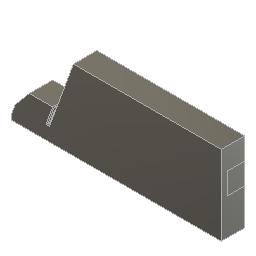
yomamamapHolder v6 (Autodesk Fusion 360 design; units mm, degrees)
Autodesk Fusion 360 part; units mm, degrees
sketch "Sketch1" plane through (0, 0, 0) normal (0, 0, 1) x (1, 0, 0)
  line L0 (0, 0) -> (12.2417, 33.6337)
  line L1 (0, 0) -> (48.7528, 0) construction
  line L2 (0, 0) -> (79.9419, 0)
  line L3 (0, 0) -> (-15, 0)
  line L4 (-1.62, 0) -> (2.6109, 11.6242)
  line L5 (-15, 0) -> (-15, -1)
  line L6 (-15, -1) -> (79.9419, -1)
  line L7 (79.9419, -1) -> (79.9419, 0)
  line L8 (2.059, 5.657) -> (2.9619, 8.1378)
  line L9 (2.9619, 8.1378) -> (18.5044, 2.4808)
  line L10 (18.5044, 2.4808) -> (17.6015, 0)
  line L11 (17.6015, 0) -> (2.059, 5.657)
  line L12 (2.9619, 8.1378) -> (3.3039, 9.0775)
  line L13 (3.3039, 9.0775) -> (17.9068, 3.7625)
  line L14 (17.9068, 3.7625) -> (17.5647, 2.8228)
  line L15 (17.5647, 2.8228) -> (2.9619, 8.1378)
  line L16 (1.717, 4.7173) -> (14.6777, 0)
  line L17 (1.546, 4.2475) -> (-13.454, 4.2475)
  line L18 (-15, 0) -> (-13.454, 4.2475)
  line L19 (12.9419, 32.6337) -> (78.9419, 32.6337)
  line L20 (78.9419, 32.6337) -> (78.9419, 6.6337)
  line L21 (78.9419, 6.6337) -> (12.9419, 6.6337)
  line L22 (12.9419, 6.6337) -> (12.9419, 32.6337)
  line L23 (12.2417, 33.6337) -> (79.9419, 33.6337)
  line L24 (79.9419, 33.6337) -> (79.9419, 0)
  line L25 (2.6109, 11.6242) -> (-7.2642, 11.6242)
  line L26 (-7.2642, 11.6242) -> (-13.454, 4.2475)
  line L27 (-8.6415, 4.2475) -> (-3.2666, 4.2475)
  line L28 (-3.2666, 4.2475) -> (-3.2666, 0)
  line L29 (-3.2666, 0) -> (-8.6415, 0)
  line L30 (-8.6415, 0) -> (-8.6415, 4.2475)
  line L31 (-3.2666, 4.2475) -> (-0.9456, 10.6242)
  line L32 (-0.9456, 10.6242) -> (1.8734, 9.5982)
  line L33 (-12.3719, 1) -> (-13.2911, 1.7713)
  line L34 (-13.2911, 1.7713) -> (-10.5662, 5.0188)
  line L35 (-10.5662, 5.0188) -> (-9.6469, 4.2475)
  line L36 (-9.6469, 4.2475) -> (-12.3719, 1)
  line L37 (12.7419, 15.4337) -> (11.7419, 15.4337)
  line L38 (11.7419, 15.4337) -> (11.7419, 5.4337)
  line L39 (11.7419, 5.4337) -> (21.7419, 5.4337)
  line L40 (21.7419, 5.4337) -> (21.7419, 6.4337)
  line L41 (12.7419, 15.4337) -> (12.7419, 6.4337)
  line L42 (12.7419, 6.4337) -> (21.7419, 6.4337)
  line L43 (59.9419, 6.4337) -> (69.9419, 6.4337)
  line L44 (69.9419, 6.4337) -> (69.9419, 5.4337)
  line L45 (69.9419, 5.4337) -> (59.9419, 5.4337)
  line L46 (59.9419, 5.4337) -> (59.9419, 6.4337)
  line L47 (79.9419, 24.6337) -> (78.9419, 24.6337)
  line L48 (78.9419, 24.6337) -> (78.9419, 14.6337)
  line L49 (78.9419, 14.6337) -> (79.9419, 14.6337)
  line L50 (79.9419, 14.6337) -> (79.9419, 24.6337)
  line L51 (-13.1502, 1.7837) -> (-10.5538, 4.8779)
  line L52 (-10.5538, 4.8779) -> (-9.7878, 4.2351)
  line L53 (-9.7878, 4.2351) -> (-12.3842, 1.1409)
  line L54 (-12.3842, 1.1409) -> (-13.1502, 1.7837)
  line L55 (-8.5415, 0.1) -> (-8.5415, 4.1475)
  line L56 (-8.5415, 4.1475) -> (-3.3666, 4.1475)
  line L57 (-3.3666, 4.1475) -> (-3.3666, 0.1)
  line L58 (-3.3666, 0.1) -> (-8.5415, 0.1)
  line L59 (-8.5415, 4.1475) -> (-8.5415, 4.2475)
  line L60 (-3.3666, 4.1475) -> (-3.3666, 4.2475)
  line L61 (12.9419, 32.6337) -> (4.2436, 8.7355)
  line L62 (78.9419, 6.6337) -> (78.9419, 0)
  line L63 (-11.3826, 3.8903) -> (-10.6165, 3.2475)
  line L64 (70.6772, 6.4337) -> (78.6772, 6.4337)
  line L65 (78.6772, 6.4337) -> (78.6772, 5.4337)
  line L66 (78.6772, 5.4337) -> (70.6772, 5.4337)
  line L67 (70.6772, 5.4337) -> (70.6772, 6.4337)
  dimension "d1" = 70
  dimension "d3" = 15
  dimension "d5" = 16.54
  dimension "d6" = 2.64
  dimension "d8" = 1
  dimension "d9" = 15.54
  dimension "d10" = 1
  dimension "d11" = 1
  dimension "d12" = 1.5
  dimension "d13" = 1.62
  dimension "d14" = 66
  dimension "d15" = 26
  dimension "d16" = 1
  dimension "d17" = 1
  dimension "d18" = 1
  dimension "d19" = 1
  dimension "d21" = 1
  dimension "d23" = 3
  dimension "d24" = 1.2
  dimension "d25" = 160
  dimension "d26" = 20
  dimension "d29" = 0.2
  dimension "d30" = 1
  dimension "d31" = 0.2
  dimension "d32" = 1
  dimension "d33" = 10
  dimension "d34" = 10
  dimension "d35" = 10
  dimension "d36" = 1
  dimension "d37" = 0.2
  dimension "d38" = 10
  dimension "d42" = 10
  dimension "d48" = 0.1
  dimension "d49" = 0.1
  dimension "d52" = 1
  dimension "d53" = 1
  dimension "d69" = 1
  dimension "d81" = 8
  dimension "d82" = 1
  constraint horizontal L1
  constraint coincident L0.start L1.start
  constraint parallel L1 L2
  constraint parallel L1 L3
  constraint coincident L3 L4.start
  constraint parallel L0 L4
  constraint perpendicular L3 L5
  constraint perpendicular L5 L6
  constraint perpendicular L2 L7
  constraint perpendicular L8 L9
  constraint parallel L8 L10
  constraint parallel L9 L11
  constraint coincident L0 L8.end
  constraint parallel L0 L8
  constraint perpendicular L12 L13
  constraint parallel L12 L14
  constraint parallel L13 L15
  constraint coincident L0 L12.end
  constraint coincident L2 L10.end
  constraint coincident L0 L16.start
  constraint coincident L1 L16.end
  constraint parallel L11 L16
  constraint coincident L0 L17.start
  constraint parallel L3 L17
  constraint parallel L4 L18
  constraint horizontal L19
  constraint vertical L20
  constraint horizontal L21
  constraint vertical L22
  constraint horizontal L23
  constraint coincident L2 L7.end
  constraint perpendicular L2 L24
  constraint horizontal L25
  constraint collinear L7 L24
  constraint horizontal L27
  constraint vertical L28
  constraint horizontal L29
  constraint vertical L30
  constraint coincident L3 L28.end
  constraint coincident L17 L27.start
  constraint midpoint L17 L27
  constraint coincident L4 L32.end
  constraint perpendicular L4 L32
  constraint coincident L17 L27.end
  constraint collinear L13 L32
  constraint parallel L4 L31
  constraint perpendicular L33 L34
  constraint parallel L33 L35
  constraint parallel L34 L36
  constraint coincident L17 L35.end
  constraint perpendicular L22 L37
  constraint perpendicular L21 L40
  constraint perpendicular L38 L39
  constraint parallel L22 L38
  constraint perpendicular L37 L41
  constraint perpendicular L40 L42
  constraint horizontal L43
  constraint vertical L44
  constraint horizontal L45
  constraint vertical L46
  constraint coincident L27.end L28.start
  constraint horizontal L47
  constraint vertical L48
  constraint horizontal L49
  constraint vertical L50
  constraint coincident L24 L47.start
  constraint midpoint L20 L48
  constraint coincident L27 L59.end
  constraint perpendicular L27 L60
  constraint coincident L27 L60.end
  constraint coincident L13 L61.end
  constraint parallel L0 L61
  constraint coincident L2 L62.end
  constraint perpendicular L2 L62
  constraint coincident L51 L63.start
  constraint coincident L53 L63.end
  constraint perpendicular L53 L63
  constraint horizontal L64
  constraint vertical L65
  constraint horizontal L66
  constraint vertical L67
  measures "d1" angle of L0 L1
  measures "d3" distance of L0.start L3.end
  measures "d5" distance of L8.start L10.end
  measures "d6" distance of L9.end L10.end
  measures "d8" distance of L3.end L5.end
  measures "d9" distance of L12.end L13.end
  measures "d10" distance of L13.end L14.end
  measures "d11" distance of L11 L16
  measures "d12" distance of L8.start L17.start
  measures "d13" distance of L0.start L4.start
  measures "d14" distance of L19.start L19.end
  measures "d15" distance of L19.start L21.end
  measures "d16" distance of L19 L23
  measures "d17" distance of L20 L24
  measures "d18" distance of L0 L19.start
  measures "d19" distance of L13 L21.end
  measures "d21" distance of L25 L31.end
  measures "d23" distance of L31.end L32.end
  measures "d24" distance of L33.start L33.end
  measures "d25" angle of L18 L26
  measures "d26" angle of L18 L34
  measures "d29" distance of L22 L41
  measures "d30" distance of L38 L41
  measures "d31" distance of L21 L42
  measures "d32" distance of L39.end L40.end
  measures "d33" distance of L38.end L39.end
  measures "d34" distance of L37.end L38.end
  measures "d35" distance of L43.start L43.end
  measures "d36" distance of L43.start L45.end
  measures "d37" distance of L21 L43
  measures "d38" distance of L24 L44
  measures "d42" distance of L47.end L48.end
  measures "d52" distance of L3 L33.start
  measures "d53" distance of L18 L33.end
  measures "d69" distance of L17 L63.end
  measures "d81" distance of L64.start L64.end
  measures "d82" distance of L64.start L66.end
extrude "Extrude1" add sketch "Sketch1" against normal blind 1 contours L0 L3 L4 L17 | L0 L2 L16 | L2 L3 L5 L6 L7 L29 | L0 L2 L11 L16 | L3 L4 L17 L28 | L2 L9 L10 L13 L14 L21 L22 L37 L38 L39 L40 L41 L42 L61 L62 | L0 L8 L9 L10 L11 L15 | L3 L17 L27 L28 L29 L30 L55 L57 L58 L59 L60 | L2 L20 L24 L49 L62 | L3 L17 L18 L30 L33 L34 L36 | L0 L9 L12 L13 L14 L15 L38 L39 | L17 L27 L56 L59 L60 | L19 L20 L21 L22 L48 | L0 L13 L19 L20 L23 L24 L47 L61 | L55 L56 L57 L58 | L20 L24 L47 L48 L49 L50 | L17 L33 L34 L36 L51 L52 L53 L54 | L13 L38 L39 | L13 L37 L38 L39 L40 L41 L42 | L17 L51 L52 L53 L63 | L51 L53 L54 L63 | L43 L44 L45 L46 | L64 L65 L66 L67 makes body 1
extrude "Extrude2" add sketch "Sketch1" against normal blind 1 separate body contours L4 L17 L31 L32 | L4 L17 L25 L26 L27 L31 L32 L34 L35 | L17 L34 L35 L51 L52 | L17 L51 L52 makes body 2
extrude "Extrude3" add sketch "Sketch1" along normal blind 7.82 contours L4 L17 L25 L26 L27 L31 L32 L34 L35 | L17 L27 L56 L59 L60 | L55 L56 L57 L58 | L17 L34 L35 L51 L52 | L17 L51 L52 L53 L63 | L17 L51 L52 bodies 2
extrude "Extrude4" add sketch "Sketch1" along normal blind 1 from surface at 7.82 contours L4 L17 L31 L32 | L4 L17 L25 L26 L27 L31 L32 L34 L35 | L17 L34 L35 L51 L52 | L17 L51 L52 bodies 2
extrude "Extrude5" add sketch "Sketch1" along normal blind 8.82 contours L0 L3 L4 L17 | L2 L3 L5 L6 L7 L29 | L3 L4 L17 L28 | L3 L17 L18 L30 L33 L34 L36 bodies 1
extrude "Extrude6" cut 2 faces at (-11.0774, 3.165, 0) (-5.0582, 2.8316, 0) along direction (0, 0, -1) blind 0.1 on bodies 1 bodies 1
extrude "Extrude7" add 2 faces at (-11.0774, 3.165, -0.1) (-5.0582, 2.8316, -0.1) along direction (0, 0, -1) blind 0.9 start surface through (0, 0, 8.82) normal (0, 0, 1) on bodies 1 bodies 1
extrude "Extrude8" add sketch "Sketch1" along normal blind 8.82 contours L0 L2 L16 | L0 L2 L11 L16 | L2 L20 L24 L49 L62 | L0 L9 L12 L13 L14 L15 L38 L39 | L0 L13 L19 L20 L23 L24 L47 L61 | L13 L38 L39 | L13 L37 L38 L39 L40 L41 L42 | L43 L44 L45 L46 | L64 L65 L66 L67 bodies 1
extrude "Extrude9" add sketch "Sketch1" against normal blind 1 from surface at 8.82 contours L0 L8 L9 L10 L11 L15 bodies 1
sketch "Sketch2" plane through (0, 0, -1) normal (0, 0, -1) x (-1, 0, 0)
  line L0 (15, -1) -> (15, 0)
  line L1 (15, 0) -> (13.454, 4.2475)
  line L2 (13.454, 4.2475) -> (-1.546, 4.2475)
  line L3 (-1.546, 4.2475) -> (-12.2417, 33.6337)
  line L4 (-12.2417, 33.6337) -> (-79.9419, 33.6337)
  line L5 (-79.9419, 33.6337) -> (-79.9419, -1)
  line L6 (-79.9419, -1) -> (15, -1)
  line L7 (-2.6109, 11.6242) -> (0.074, 4.2475)
  line L8 (0.074, 4.2475) -> (13.454, 4.2475)
  line L9 (13.454, 4.2475) -> (7.2642, 11.6242)
  line L10 (7.2642, 11.6242) -> (-2.6109, 11.6242)
  line L11 (-80.0419, -1.1) -> (15.1, -1.1)
  line L12 (15.1, -1.1) -> (15.1, 0.0176)
  line L13 (15.1, 0.0176) -> (13.542, 4.2982)
  line L14 (13.5007, 4.3475) -> (-1.4759, 4.3475)
  line L15 (-12.2781, 33.7337) -> (-80.0419, 33.7337)
  line L16 (-80.0419, 33.7337) -> (-80.0419, -1.1)
  line L17 (13.4904, 4.1475) -> (13.5969, 4.1475)
  line L18 (13.542, 4.2982) -> (7.3109, 11.7242)
  line L19 (7.3109, 11.7242) -> (-2.6473, 11.7242)
  line L20 (-0.0688, 4.3475) -> (-0.0324, 4.2475)
  line L21 (-2.6109, 11.6242) -> (-2.6473, 11.7242)
  line L22 (-12.2417, 33.6337) -> (-12.2781, 33.7337)
  line L23 (-12.2781, 34.7337) -> (-81.0419, 34.7337)
  line L24 (-81.0419, 34.7337) -> (-81.0419, -2.1)
  line L25 (-81.0419, -2.1) -> (16.1, -2.1)
  line L26 (16.1, -2.1) -> (16.1, 0.194)
  line L27 (16.1, 0.194) -> (14.4214, 4.806)
  line L28 (14.4214, 4.806) -> (7.7772, 12.7242)
  line L29 (7.7772, 12.7242) -> (-2.6473, 12.7242)
  line L30 (-12.2417, 33.6337) -> (-12.642, 34.7337)
  line L31 (-2.6473, 11.7242) -> (-3.0112, 12.7242)
  line L32 (-3.0112, 12.7242) -> (-2.6473, 12.7242)
  line L33 (-80.0419, 14.6337) -> (-81.0419, 14.6337)
  line L34 (-80.0419, 24.6337) -> (-81.0419, 24.6337)
  line L35 (-78.9419, 24.6337) -> (-79.9419, 24.6337)
  line L36 (-79.9419, 14.6337) -> (-78.9419, 14.6337)
  dimension "d73" = 1
  constraint coincident L1 L17.start
  constraint coincident L2 L20.end
  constraint coincident L14 L20.start
  constraint coincident L7.start L10.end
  constraint coincident L19 L21.end
  constraint parallel L7 L21
  constraint coincident L19.end L21
  constraint coincident L3.end L4.start
  constraint coincident L15 L22.end
  constraint collinear L3 L22
  constraint coincident L15.start L22
  constraint coincident L13 L17.end
  constraint coincident L18 L14.start
  constraint coincident L23 L30.end
  constraint collinear L3 L30
  constraint coincident L29 L31.end
  constraint collinear L7 L31
  constraint coincident L16 L33.start
  constraint coincident L24 L33.end
  constraint perpendicular L24 L33
  constraint coincident L16 L34.start
  constraint coincident L24 L34.end
  constraint perpendicular L24 L34
  constraint collinear L34 L35
  constraint collinear L33 L36
extrude "Extrude10" add sketch "Sketch2" against normal blind 9.82 separate body contours L11 L12 L13 L16 L18 L19 L24 L25 L26 L27 L28 L29 L31 L32 L33 | L15 L16 L23 L24 L30 L34 | L16 L24 L33 L34 makes body 3
extrude "Extrude11" add sketch "Sketch2" against normal blind 1 from surface at -9.82 contours L0 L1 L2 L3 L4 L5 L6 L8 | L0 L1 L4 L5 L6 L11 L12 L13 L15 L16 L17 L22 L30 | L1 L9 L13 L14 L17 L18 | L2 L7 L8 L9 L14 | L11 L12 L13 L16 L18 L19 L24 L25 L26 L27 L28 L29 L31 L32 L33 | L7 L9 L10 L14 | L9 L10 L14 L18 L19 L21 | L15 L16 L23 L24 L30 L34 | L16 L24 L33 L34 bodies 3
extrude "Extrude13" cut sketch "Sketch2" against normal blind 8 contours L16 L24 L33 L34 bodies 3
extrude "Extrude12" add sketch "Sketch2" against normal blind 10.82 separate body contours L0 L1 L2 L3 L4 L5 L6 L8 | L0 L1 L4 L5 L6 L11 L12 L13 L15 L16 L17 L22 L30 | L1 L9 L13 L14 L17 L18 | L2 L7 L8 L9 L14 | L11 L12 L13 L16 L18 L19 L24 L25 L26 L27 L28 L29 L31 L32 L33 | L7 L9 L10 L14 | L9 L10 L14 L18 L19 L21 | L15 L16 L23 L24 L30 L34 | L16 L24 L33 L34 makes body 4
equation "d5 = dupont_l"
equation "d6 = 2.54 mm + off"
equation "off = 0.1 mm" comment "offset dupont (clearance)"
equation "d8 = stena"
equation "d9 = d5 - 1 mm"
equation "d10 = stena"
equation "d11 = stena"
equation "d14 = esp_lenght"
equation "d15 = esp_width"
equation "d16 = stena"
equation "d17 = stena"
equation "d18 = stena"
equation "d19 = stena"
equation "d21 = stena"
equation "stena = 1 mm"
equation "d24 = stena + 0.2 mm"
equation "d30 = stena"
equation "d31 = d29"
equation "d32 = stena"
equation "d36 = stena"
equation "esp_width = 26 mm"
equation "esp_lenght = 66 mm"
equation "dupont_l = 14 mm + 2.54 mm" comment "DupontSocket plus recesed pin header"
equation "d43 = -stena"
equation "d45 = -stena"
equation "dupont3width = ( 3 * 2.54 ) * 1 mm + 0.2 mm"
equation "d50 = dupont3width"
equation "d52 = stena"
equation "d53 = stena"
equation "d55 = stena"
equation "d62 = -stena + 0.1 mm"
equation "d67 = -stena"
equation "d82 = d36"
named bodies: "LeftLeg", "LeftFrontCap", "LeftLegCover", "RightLeg"
